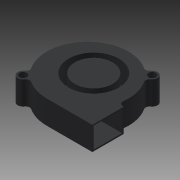
# Autodesk Inventor part: blowerFan50x15
Saved by Autodesk Inventor 2013 (Build 170138000, 138)
## iProperties
Created: 2015-01-15
Part Number: blowerFan50x15
Material: Generic
Document SubType Name: Modeling
Designer: dzban
Density: 1 g/cm^3
Author: dzban
Autodesk Inventor part; units mm, degrees
ref_plane "YZ Plane" through (0, 0, 0) normal (1, 0, 0) x (0, 1, 0)
ref_plane "XZ Plane" through (0, 0, 0) normal (0, 1, 0) x (-1, 0, 0)
ref_plane "XY Plane" through (0, 0, 0) normal (0, 0, 1) x (1, 0, 0)
sketch "Sketch1" plane through (0, 0, 0) normal (0, 0, 1) x (1, 0, 0)
  line L0 (26, 0) -> (52, 0)
  circle A0 centre (46.5768, 46.5768) radius 2.4
  arc A1 (48.4457, 43.7365) -> (43.7365, 48.4457) centre (46.5768, 46.5768) ccw
  arc A2 (3.5543, 8.2635) -> (8.2635, 3.5543) centre (5.4232, 5.4232) ccw
  circle A3 centre (5.4232, 5.4232) radius 2.4
  line L1 (55, 0) -> (55, 20)
  arc A4 (40.2754, 47.7304) -> (43.7365, 48.4457) centre (41.6481, 49.8199) ccw
  arc A5 (48.4457, 43.7365) -> (47.7304, 40.2754) centre (49.8199, 41.6481) ccw
  arc A6 (40.2754, 47.7304) -> (4.2696, 11.7246) centre (26, 26) ccw
  arc A7 (11.7246, 4.2696) -> (8.2635, 3.5543) centre (10.3519, 2.1801) ccw
  arc A8 (3.5543, 8.2635) -> (4.2696, 11.7246) centre (2.1801, 10.3519) ccw
  arc A9 (11.7246, 4.2696) -> (26, 0) centre (26, 26) ccw
  arc A10 (51.8032, 22.807) -> (47.7304, 40.2754) centre (26, 26) ccw
  arc A11 (51.8032, 22.807) -> (54.2843, 20) centre (54.2843, 22.5) ccw
  line L2 (55, 0) -> (52, 0)
  line L3 (55, 20) -> (54.2843, 20)
  point P0 (48.981, 48.981)
  dimension "d6" = 4.8
  dimension "d7" = 29
  dimension "d8" = 20
  dimension "d9" = 2.5
  dimension "d10" = 2.5
  dimension "d11" = 2.5
  constraints: 21 point on circle, 12 centre point, 8 end point, 6 tangent, 2 coincident, 2 equal radius, 1 horizontal, 1 point on line, 2 other
  measures "d6" diameter of A0
  measures "d7" distance of L0.start L1.start
  measures "d8" distance of L1.start L1.end
  measures "d9" radius of A4
  measures "d10" radius of A7
  measures "d11" radius of A11
extrude "Extrusion1" add sketch "Sketch1" along normal blind 15
sketch "Sketch2" plane through (55, 0, 0) normal (1, 0, 0) x (0, 0, -1)
  line L0 (-14.1994, 18.9903) -> (-0.92, 18.9903)
  line L1 (-0.92, 18.9903) -> (-0.92, 0.7311)
  line L2 (-0.92, 0.7311) -> (-14.1994, 0.7311)
  line L3 (-14.1994, 0.7311) -> (-14.1994, 18.9903)
  constraints: 8 end point
extrude "Extrusion2" cut sketch "Sketch2" against normal blind 15
sketch "Sketch3" plane through (0, 0, 15) normal (0, 0, 1) x (1, 0, 0)
  circle A0 centre (26.8751, 29.0108) radius 12
  circle A1 centre (26.8751, 29.0108) radius 16
  point P0 (0, 0)
  dimension "d16" = 24
  dimension "d18" = 32
  constraints: 2 centre point, 1 coincident
  measures "d16" diameter of A0
  measures "d18" diameter of A1
extrude "Extrusion3" cut sketch "Sketch3" against normal blind 14
body "Solid1"
